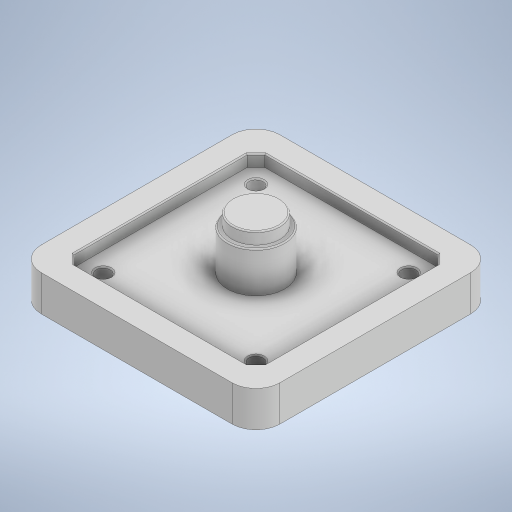
# Autodesk Inventor part: Base1
Saved by Autodesk Inventor 2024.2 (Build 282272000, 272)
## iProperties
Created: 2024-04-19
Part Number: Base1
Material: Generic
Document SubType Name: Modeling
Designer: 062210026
Density: 1 g/cm^3
Appearance: Default
Author: 062210026
Autodesk Inventor part; units mm, degrees
ref_plane "YZ Plane" through (0, 0, 0) normal (1, 0, 0) x (0, 1, 0)
ref_plane "XZ Plane" through (0, 0, 0) normal (0, 1, 0) x (-1, 0, 0)
ref_plane "XY Plane" through (0, 0, 0) normal (0, 0, 1) x (1, 0, 0)
sketch "Sketch1" plane through (0, 0, 0) normal (0, 1, 0) x (-1, 0, 0)
  line L0 (40, 50) -> (-40, 50)
  line L1 (-50, 40) -> (-50, -40)
  line L2 (-40, -50) -> (40, -50)
  line L3 (50, -40) -> (50, 40)
  line L4 (50, 50) -> (-50, -50) construction
  line L5 (-50, 50) -> (50, -50) construction
  arc A0 (-40, 50) -> (-50, 40) centre (-40, 40) ccw
  arc A1 (50, 40) -> (40, 50) centre (40, 40) ccw
  arc A2 (-50, -40) -> (-40, -50) centre (-40, -40) ccw
  arc A3 (40, -50) -> (50, -40) centre (40, -40) ccw
  point P0 (0, 0)
  dimension "d0" = 100
  dimension "d1" = 100
  dimension "d2" = 10
  dimension "d3" = 10
  dimension "d4" = 10
  constraints: 12 end point, 8 point on circle, 8 point on line, 8 tangent, 4 centre point, 2 midpoint, 2 parallel, 1 equal radius, 1 horizontal, 1 perpendicular
  measures "d0" distance of L5.end L4.end
  measures "d1" distance of L5.end L4.start
  measures "d2" radius of A0
  measures "d3" radius of A1
  measures "d4" radius of A2
extrude "Extrusion1" add sketch "Sketch1" along normal blind 15
sketch "Sketch2" plane through (0, 15, 0) normal (0, 1, 0) x (1, 0, 0)
  line L0 (-36.2734, -40) -> (36.2734, -40)
  line L1 (40, -36.2734) -> (40, 36.2734)
  line L2 (36.2734, 40) -> (-36.2734, 40)
  line L3 (-40, 36.2734) -> (-40, -36.2734)
  line L4 (-40, -40) -> (40, 40) construction
  line L5 (40, -40) -> (-40, 40) construction
  line L6 (-36.2734, -40) -> (-40, -36.2734)
  line L7 (-36.2734, 40) -> (-40, 36.2734)
  line L8 (36.2734, -40) -> (40, -36.2734)
  line L9 (36.2734, 40) -> (40, 36.2734)
  point P0 (0, 0)
  dimension "d7" = 80
  dimension "d8" = 80
  dimension "d9" = 3.7266
  dimension "d10" = 3.7266
  dimension "d11" = 3.7266
  dimension "d12" = 3.7266
  dimension "d13" = 3.7266
  dimension "d14" = 3.7266
  dimension "d15" = 3.7266
  dimension "d16" = 3.7266
  constraints: 20 end point, 8 point on line, 2 midpoint, 2 parallel, 1 horizontal, 1 perpendicular
  measures "d7" distance of L5.end L4.end
  measures "d8" distance of L4.end L5.start
  measures "d9" distance of L0.start L4.start
  measures "d10" distance of L3.end L4.start
  measures "d11" distance of L2.end L5.end
  measures "d12" distance of L3.start L5.end
  measures "d13" distance of L0.end L5.start
  measures "d14" distance of L1.start L5.start
  measures "d15" distance of L2.start L4.end
  measures "d16" distance of L1.end L4.end
extrude "Extrusion2" cut sketch "Sketch2" against normal blind 5
sketch "Sketch3" plane through (0, 10, 0) normal (0, 1, 0) x (1, 0, 0)
  line L0 (0, 0) -> (32, 0)
  line L1 (32, 0) -> (32, -32)
  circle A0 centre (32, -32) radius 3
  circle A1 centre (32, 32) radius 3
  circle A2 centre (-32, 32) radius 3
  circle A3 centre (-32, -32) radius 3
  dimension "d19" = 32
  dimension "d20" = 32
  dimension "d21" = 6
  dimension "d24" = 360
  constraints: 4 centre point, 4 end point, 1 coincident, 1 horizontal, 1 perpendicular, 9 other
  measures "d19" distance of L0.start L0.end
  measures "d20" distance of L0.end L1.end
  measures "d21" diameter of A0
extrude "Extrusion3" cut sketch "Sketch3" against normal blind 20
sketch "Sketch4" plane through (0, 10, 0) normal (0, 1, 0) x (1, 0, 0)
  circle A0 centre (0, 0) radius 12
  dimension "d28" = 24
  constraints: 1 centre point, 1 coincident
  measures "d28" diameter of A0
extrude "Extrusion4" add sketch "Sketch4" along normal blind 17
sketch "Sketch5" plane through (0, 27, 0) normal (0, 1, 0) x (1, 0, 0)
  circle A0 centre (0, 0) radius 10
  dimension "d31" = 20
  constraints: 1 centre point, 1 coincident
  measures "d31" diameter of A0
extrude "Extrusion5" add sketch "Sketch5" along normal blind 5
fillet "Fillet1" radius 0.5 2 edges at (-12, 27, 0) (-10, 32, 0)
chamfer "Chamfer1" distance 0.5 angle 45 12 edges at (-35, 10, 32) (29, 10, 32) (29, 10, -32) (-35, 10, -32) (0, 15, 40) (-38.1367, 15, 38.1367) (-40, 15, 0) (-38.1367, 15, -38.1367) (0, 15, -40) (38.1367, 15, -38.1367) (40, 15, 0) (38.1367, 15, 38.1367)
equation "\"d0\" = d1"
equation "\"d8\" = d7"
equation "\"d10\" = d9"
equation "\"d11\" = d9"
equation "\"d12\" = d9"
equation "\"d13\" = d9"
equation "\"d14\" = d9"
equation "\"d15\" = d9"
equation "\"d16\" = d9"
body "Solid1"
